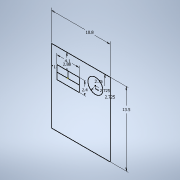
# Autodesk Inventor part: VL53LDK
Saved by Autodesk Inventor 2022 (Build 260153070, 153G)
## iProperties
Created: 2022-01-11
Part Number: VL53LDK
Material: Generic
Document SubType Name: Modeling
Designer: a laptop
Density: 1 g/cm^3
Appearance: Default
Author: a laptop
Autodesk Inventor part; units mm, degrees
ref_plane "YZ Plane" through (0, 0, 0) normal (1, 0, 0) x (0, 1, 0)
ref_plane "XZ Plane" through (0, 0, 0) normal (0, 1, 0) x (-1, 0, 0)
ref_plane "XY Plane" through (0, 0, 0) normal (0, 0, 1) x (1, 0, 0)
sketch "Sketch1" plane through (0, 0, 0) normal (0, 0, 1) x (1, 0, 0)
  line L0 (-3.05, 4.08) -> (7.75, 4.08)
  line L1 (7.75, 4.08) -> (7.75, -9.42)
  line L2 (7.75, -9.42) -> (-3.05, -9.42)
  line L3 (-3.05, -9.42) -> (-3.05, 4.08)
  circle A0 centre (5.025, 1.355) radius 1.375
  line L4 (-2.05, 1.2) -> (2.05, 1.2)
  line L5 (2.05, 1.2) -> (2.05, -1.2)
  line L6 (2.05, -1.2) -> (-2.05, -1.2)
  line L7 (-2.05, -1.2) -> (-2.05, 1.2)
  line L8 (-2.05, 0) -> (2.05, 0)
  line L9 (0, 1.2) -> (0, 0)
  dimension "d0" = 10.8
  dimension "d1" = 13.5
  dimension "d2" = 2.725
  dimension "d3" = 2.725
  dimension "d4" = 2.75
  dimension "d5" = 4.1
  dimension "d6" = 2.4
  dimension "d7" = 1
  dimension "d8" = 2.88
  constraints: 20 end point, 4 midpoint, 4 parallel, 2 horizontal, 2 perpendicular, 1 centre point, 1 coincident
  measures "d0" distance of L0.start L0.end
  measures "d1" distance of L0.end L1.end
  measures "d2" distance from line of L1 A0.centre
  measures "d3" distance from line of L0 A0.centre
  measures "d4" diameter of A0
  measures "d5" distance of L4.start L4.end
  measures "d6" distance of L4.end L5.end
  measures "d7" distance between parallel lines of L3 L7
  measures "d8" distance between parallel lines of L4 L0
extrude "Extrusion1" add sketch "Sketch1" along normal blind 1.65
extrude "Extrusion2" add sketch "Sketch1" along normal blind 2.75 contours L4 L9 L8 L7 | L4 L5 L8 L9 | L8 L5 L6 L7
body "Solid1"
